Autodesk Inventor part; units mm, degrees
(part 2 of 2)
  line L687 (11.384, -26.5017) -> (12.8968, -23.7765)
  line L688 (8.2674, -26.5542) -> (11.384, -26.5017)
  line L689 (24.5423, -12.481) -> (26.7401, -16.1439)
  line L690 (24.5423, -12.481) -> (20.2713, -12.5528)
  line L691 (24.6668, -19.8787) -> (26.7401, -16.1439)
  line L692 (24.6668, -19.8787) -> (20.3957, -19.9505)
  line L693 (25.5855, -16.1633) -> (24.0727, -18.8885)
  line L694 (24.0727, -18.8885) -> (20.9562, -18.9409)
  line L695 (23.9819, -13.4905) -> (25.5855, -16.1633)
  line L696 (19.3525, -16.2682) -> (20.8654, -13.543)
  line L697 (20.8654, -13.543) -> (23.9819, -13.4905)
  line L698 (20.9562, -18.9409) -> (19.3525, -16.2682)
  line L699 (18.198, -16.2876) -> (20.3957, -19.9505)
  line L700 (20.5202, -27.3482) -> (24.7912, -27.2763)
  line L701 (20.5202, -27.3482) -> (18.3224, -23.6853)
  line L702 (19.4769, -23.6659) -> (21.0806, -26.3386)
  line L703 (20.9898, -20.9407) -> (19.4769, -23.6659)
  line L704 (18.3224, -23.6853) -> (20.3957, -19.9505)
  line L705 (24.1063, -20.8882) -> (20.9898, -20.9407)
  line L706 (25.71, -23.561) -> (24.1063, -20.8882)
  line L707 (24.6668, -19.8787) -> (26.8645, -23.5416)
  line L708 (24.7912, -27.2763) -> (26.8645, -23.5416)
  line L709 (24.1971, -26.2862) -> (25.71, -23.561)
  line L710 (21.0806, -26.3386) -> (24.1971, -26.2862)
  line L711 (30.8867, -8.6744) -> (33.0844, -12.3373)
  line L712 (30.8867, -8.6744) -> (26.6156, -8.7462)
  line L713 (31.0111, -16.072) -> (33.0844, -12.3373)
  line L714 (30.3262, -9.6839) -> (27.2097, -9.7364)
  line L715 (30.3262, -9.6839) -> (31.9299, -12.3567)
  line L716 (30.417, -15.0819) -> (31.9299, -12.3567)
  line L717 (31.0111, -16.072) -> (26.7401, -16.1439)
  line L718 (27.3005, -15.1343) -> (30.417, -15.0819)
  line L719 (26.7401, -16.1439) -> (24.5423, -12.481)
  line L720 (25.6969, -12.4616) -> (27.3005, -15.1343)
  line L721 (25.6969, -12.4616) -> (27.2097, -9.7364)
  line L722 (24.6668, -19.8787) -> (26.8645, -23.5416)
  line L723 (24.6668, -19.8787) -> (26.7401, -16.1439)
  line L724 (25.8213, -19.8592) -> (27.425, -22.532)
  line L725 (25.8213, -19.8592) -> (27.3342, -17.134)
  line L726 (27.3342, -17.134) -> (30.4507, -17.0816)
  line L727 (30.4507, -17.0816) -> (32.0543, -19.7544)
  line L728 (31.0111, -16.072) -> (33.2089, -19.735)
  line L729 (31.1356, -23.4697) -> (33.2089, -19.735)
  line L730 (30.5415, -22.4796) -> (32.0543, -19.7544)
  line L731 (30.5415, -22.4796) -> (27.425, -22.532)
  line L732 (31.1356, -23.4697) -> (26.8645, -23.5416)
  line L733 (37.231, -4.8677) -> (32.96, -4.9396)
  line L734 (37.231, -4.8677) -> (39.4288, -8.5307)
  line L735 (36.6706, -5.8773) -> (38.2742, -8.5501)
  line L736 (36.7614, -11.2753) -> (38.2742, -8.5501)
  line L737 (39.4288, -8.5307) -> (37.3555, -12.2654)
  line L738 (32.0412, -8.6549) -> (33.6449, -11.3277)
  line L739 (33.5541, -5.9297) -> (36.6706, -5.8773)
  line L740 (32.0412, -8.6549) -> (33.5541, -5.9297)
  line L741 (36.7614, -11.2753) -> (33.6449, -11.3277)
  line L742 (37.3555, -12.2654) -> (33.0844, -12.3373)
  line L743 (30.8867, -8.6744) -> (33.0844, -12.3373)
  line L744 (37.4799, -19.6631) -> (39.5532, -15.9283)
  line L745 (37.4799, -19.6631) -> (33.2089, -19.735)
  line L746 (36.8858, -18.673) -> (38.3987, -15.9478)
  line L747 (36.8858, -18.673) -> (33.7693, -18.7254)
  line L748 (33.7693, -18.7254) -> (32.1657, -16.0526)
  line L749 (31.0111, -16.072) -> (33.2089, -19.735)
  line L750 (32.1657, -16.0526) -> (33.6785, -13.3274)
  line L751 (37.3555, -12.2654) -> (33.0844, -12.3373)
  line L752 (36.795, -13.275) -> (33.6785, -13.3274)
  line L753 (36.795, -13.275) -> (38.3987, -15.9478)
  line L754 (37.3555, -12.2654) -> (39.5532, -15.9283)
  line L755 (31.1356, -23.4697) -> (33.3333, -27.1326)
  line L756 (37.6044, -27.0608) -> (33.3333, -27.1326)
  line L757 (32.2901, -23.4503) -> (33.8938, -26.1231)
  line L758 (33.803, -20.7251) -> (32.2901, -23.4503)
  line L759 (31.1356, -23.4697) -> (33.2089, -19.735)
  line L760 (36.9195, -20.6727) -> (33.803, -20.7251)
  line L761 (36.9195, -20.6727) -> (38.5231, -23.3455)
  line L762 (37.4799, -19.6631) -> (39.6777, -23.326)
  line L763 (37.6044, -27.0608) -> (39.6777, -23.326)
  line L764 (37.0103, -26.0706) -> (38.5231, -23.3455)
  line L765 (37.0103, -26.0706) -> (33.8938, -26.1231)
  line L766 (45.8976, -12.1217) -> (43.6998, -8.4588)
  line L767 (45.8976, -12.1217) -> (43.8243, -15.8565)
  line L768 (43.8243, -15.8565) -> (39.5532, -15.9283)
  line L769 (43.2302, -14.8663) -> (44.743, -12.1412)
  line L770 (43.2302, -14.8663) -> (40.1137, -14.9188)
  line L771 (38.51, -12.246) -> (40.1137, -14.9188)
  line L772 (37.3555, -12.2654) -> (39.5532, -15.9283)
  line L773 (38.51, -12.246) -> (40.0229, -9.5208)
  line L774 (43.6998, -8.4588) -> (39.4288, -8.5307)
  line L775 (43.1394, -9.4684) -> (40.0229, -9.5208)
  line L776 (44.743, -12.1412) -> (43.1394, -9.4684)
  line L777 (43.6998, -8.4588) -> (45.8976, -12.1217)
  line L778 (43.9487, -23.2542) -> (39.6777, -23.326)
  line L779 (39.6777, -23.326) -> (37.4799, -19.6631)
  line L780 (37.4799, -19.6631) -> (39.5532, -15.9283)
  line L781 (38.6345, -19.6437) -> (40.2381, -22.3165)
  line L782 (38.6345, -19.6437) -> (40.1473, -16.9185)
  line L783 (43.2638, -16.8661) -> (40.1473, -16.9185)
  line L784 (43.2638, -16.8661) -> (44.8675, -19.5388)
  line L785 (46.022, -19.5194) -> (43.8243, -15.8565)
  line L786 (43.9487, -23.2542) -> (46.022, -19.5194)
  line L787 (44.8675, -19.5388) -> (43.3546, -22.264)
  line L788 (43.3546, -22.264) -> (40.2381, -22.3165)
  line L789 (50.1686, -12.0499) -> (52.2419, -8.3151)
  line L790 (52.2419, -8.3151) -> (50.0442, -4.6522)
  line L791 (49.5745, -11.0597) -> (51.0874, -8.3345)
  line L792 (49.4837, -5.6618) -> (51.0874, -8.3345)
  line L793 (45.7731, -4.724) -> (50.0442, -4.6522)
  line L794 (49.4837, -5.6618) -> (46.3672, -5.7142)
  line L795 (44.8544, -8.4394) -> (46.3672, -5.7142)
  line L796 (46.458, -11.1122) -> (44.8544, -8.4394)
  line L797 (43.6998, -8.4588) -> (45.8976, -12.1217)
  line L798 (49.5745, -11.0597) -> (46.458, -11.1122)
  line L799 (45.8976, -12.1217) -> (50.1686, -12.0499)
  line L800 (46.022, -19.5194) -> (50.2931, -19.4476)
  line L801 (46.022, -19.5194) -> (43.8243, -15.8565)
  line L802 (43.8243, -15.8565) -> (45.8976, -12.1217)
  line L803 (44.9788, -15.8371) -> (46.5825, -18.5098)
  line L804 (46.4917, -13.1119) -> (44.9788, -15.8371)
  line L805 (49.6082, -13.0595) -> (46.4917, -13.1119)
  line L806 (49.6082, -13.0595) -> (51.2119, -15.7322)
  line L807 (50.1686, -12.0499) -> (52.3664, -15.7128)
  line L808 (52.3664, -15.7128) -> (50.2931, -19.4476)
  line L809 (49.699, -18.4574) -> (51.2119, -15.7322)
  line L810 (49.699, -18.4574) -> (46.5825, -18.5098)
  line L811 (46.1465, -26.9171) -> (43.9487, -23.2542)
  line L812 (46.022, -19.5194) -> (43.9487, -23.2542)
  line L813 (46.1465, -26.9171) -> (50.4175, -26.8452)
  line L814 (49.7326, -20.4571) -> (46.6161, -20.5096)
  line L815 (45.1033, -23.2348) -> (46.6161, -20.5096)
  line L816 (46.7069, -25.9075) -> (45.1033, -23.2348)
  line L817 (49.8234, -25.8551) -> (46.7069, -25.9075)
  line L818 (49.8234, -25.8551) -> (51.3363, -23.1299)
  line L819 (50.4175, -26.8452) -> (52.4908, -23.1105)
  line L820 (49.7326, -20.4571) -> (51.3363, -23.1299)
  line L821 (52.4908, -23.1105) -> (50.2931, -19.4476)
  line L822 (50.2931, -19.4476) -> (52.4908, -23.1105)
  line L823 (50.1686, -12.0499) -> (52.2419, -8.3151)
  line L824 (52.2419, -8.3151) -> (50.0442, -4.6522)
  line L825 (52.8024, -7.3055) -> (55.9189, -7.2531)
  line L826 (56.513, -8.2433) -> (52.2419, -8.3151)
  line L827 (52.8024, -7.3055) -> (51.1987, -4.6328)
  line L828 (52.836, -9.3053) -> (51.3232, -12.0305)
  line L829 (55.9525, -9.2528) -> (52.836, -9.3053)
  line L830 (57.5562, -11.9256) -> (55.9525, -9.2528)
  line L831 (56.513, -8.2433) -> (58.7107, -11.9062)
  line L832 (51.3232, -12.0305) -> (52.9268, -14.7032)
  line L833 (50.1686, -12.0499) -> (52.3664, -15.7128)
  line L834 (56.0434, -14.6508) -> (57.5562, -11.9256)
  line L835 (56.6374, -15.6409) -> (58.7107, -11.9062)
  line L836 (56.6374, -15.6409) -> (58.7107, -11.9062)
  line L837 (52.9605, -16.7029) -> (51.4476, -19.4281)
  line L838 (52.3664, -15.7128) -> (50.2931, -19.4476)
  line L839 (56.077, -16.6505) -> (52.9605, -16.7029)
  line L840 (52.9268, -14.7032) -> (56.0434, -14.6508)
  line L841 (56.6374, -15.6409) -> (52.3664, -15.7128)
  line L842 (51.4476, -19.4281) -> (53.0513, -22.1009)
  line L843 (57.6807, -19.3233) -> (56.077, -16.6505)
  line L844 (58.8352, -19.3039) -> (56.6374, -15.6409)
  line L845 (56.1678, -22.0485) -> (57.6807, -19.3233)
  line L846 (56.7619, -23.0386) -> (58.8352, -19.3039)
  line L847 (53.0513, -22.1009) -> (56.1678, -22.0485)
  line L848 (56.513, -8.2433) -> (58.5863, -4.5085)
  line L849 (55.9189, -7.2531) -> (57.4318, -4.5279)
  line L850 (58.5863, -4.5085) -> (56.3885, -0.8456)
  line L851 (57.4318, -4.5279) -> (55.8281, -1.8552)
  line L852 (52.7116, -1.9076) -> (55.8281, -1.8552)
  line L853 (51.1987, -4.6328) -> (52.7116, -1.9076)
  line L854 (50.0442, -4.6522) -> (52.1175, -0.9174)
  line L855 (56.7619, -23.0386) -> (52.4908, -23.1105)
  line L856 (59.2712, -10.8966) -> (57.6675, -8.2238)
  line L857 (56.513, -8.2433) -> (58.7107, -11.9062)
  line L858 (62.4214, -12.8439) -> (59.3048, -12.8963)
  line L859 (58.7107, -11.9062) -> (62.9205, -11.8718)
  line L860 (62.3877, -10.8442) -> (59.2712, -10.8966)
  line L861 (64.1363, -11.8149) -> (65.74, -14.4877)
  line L862 (64.025, -15.5167) -> (62.4214, -12.8439)
  line L863 (62.9205, -11.8718) -> (65.1795, -15.4973)
  line L864 (56.6374, -15.6409) -> (58.7107, -11.9062)
  line L865 (59.3048, -12.8963) -> (57.792, -15.6215)
  line L866 (62.5122, -18.2419) -> (64.025, -15.5167)
  line L867 (59.3956, -18.2943) -> (62.5122, -18.2419)
  line L868 (63.1062, -19.232) -> (58.8352, -19.3039)
  line L869 (57.792, -15.6215) -> (59.3956, -18.2943)
  line L870 (65.1795, -15.4973) -> (63.1062, -19.232)
  line L871 (58.8352, -19.3039) -> (56.6374, -15.6409)
  line L872 (56.7619, -23.0386) -> (58.8352, -19.3039)
  line L873 (69.4506, -15.4254) -> (65.1795, -15.4973)
  line L874 (68.8565, -14.4353) -> (65.74, -14.4877)
  line L875 (64.1363, -11.8149) -> (65.6492, -9.0897)
  line L876 (65.6492, -9.0897) -> (68.7657, -9.0373)
  line L877 (70.3694, -11.7101) -> (68.7657, -9.0373)
  line L878 (68.8565, -14.4353) -> (70.3694, -11.7101)
  line L879 (71.5239, -11.6906) -> (69.4506, -15.4254)
  line L880 (69.3262, -8.0277) -> (71.5239, -11.6906)
  line L881 (69.3262, -8.0277) -> (65.0551, -8.0996)
  line L882 (63.9006, -8.119) -> (62.3877, -10.8442)
  line L883 (65.0551, -8.0996) -> (62.8574, -4.4367)
  line L884 (62.2969, -5.4462) -> (63.9006, -8.119)
  line L885 (62.8574, -4.4367) -> (58.5863, -4.5085)
  line L886 (59.1804, -5.4986) -> (62.2969, -5.4462)
  line L887 (57.6675, -8.2238) -> (59.1804, -5.4986)
  line L888 (56.513, -8.2433) -> (58.5863, -4.5085)
  line L889 (58.9596, -26.7015) -> (56.7619, -23.0386)
  line L890 (58.9596, -26.7015) -> (63.2307, -26.6297)
  line L891 (59.4293, -20.294) -> (62.5458, -20.2416)
  line L892 (57.9164, -23.0192) -> (59.4293, -20.294)
  line L893 (59.5201, -25.692) -> (57.9164, -23.0192)
  line L894 (64.1495, -22.9144) -> (62.6366, -25.6396)
  line L895 (62.6366, -25.6396) -> (59.5201, -25.692)
  line L896 (62.5458, -20.2416) -> (64.1495, -22.9144)
  line L897 (63.1062, -19.232) -> (65.304, -22.8949)
  line L898 (68.6413, -1.6396) -> (70.2449, -4.3124)
  line L899 (70.2449, -4.3124) -> (68.7321, -7.0376)
  line L900 (69.3262, -8.0277) -> (71.3995, -4.293)
  line L901 (65.6156, -7.09) -> (68.7321, -7.0376)
  line L902 (64.0119, -4.4172) -> (65.6156, -7.09)
  line L903 (65.0551, -8.0996) -> (62.8574, -4.4367)
  line L904 (64.0119, -4.4172) -> (65.5247, -1.692)
  line L905 (62.8574, -4.4367) -> (64.9307, -0.7019)
  line L906 (68.6413, -1.6396) -> (65.5247, -1.692)
  line L907 (71.3995, -4.293) -> (69.2017, -0.63)
  line L908 (65.8644, -21.8854) -> (68.981, -21.8329)
  line L909 (69.575, -22.8231) -> (65.304, -22.8949)
  line L910 (64.2608, -19.2126) -> (65.8644, -21.8854)
  line L911 (65.304, -22.8949) -> (63.1062, -19.232)
  line L912 (63.1062, -19.232) -> (65.1795, -15.4973)
  line L913 (64.2608, -19.2126) -> (65.7736, -16.4874)
  line L914 (68.8902, -16.435) -> (65.7736, -16.4874)
  line L915 (71.6484, -19.0883) -> (69.4506, -15.4254)
  line L916 (68.8902, -16.435) -> (70.4938, -19.1077)
  line L917 (70.4938, -19.1077) -> (68.981, -21.8329)
  line L918 (69.575, -22.8231) -> (71.6484, -19.0883)
  line L919 (65.8981, -23.8851) -> (69.0146, -23.8327)
  line L920 (63.2307, -26.6297) -> (65.304, -22.8949)
  line L921 (62.9205, -11.8718) -> (65.0551, -8.0996)
  line L922 (59.1467, -3.4989) -> (57.5431, -0.8262)
  line L923 (56.3885, -0.8456) -> (58.5863, -4.5085)
  line L924 (58.5863, -4.5085) -> (62.8574, -4.4367)
  line L925 (62.2633, -3.4465) -> (59.1467, -3.4989)
  line L926 (64.9307, -0.7019) -> (62.8574, -4.4367)
  line L927 (63.7761, -0.7213) -> (62.2633, -3.4465)
  line L928 (64.9307, -0.7019) -> (62.7329, 2.961)
  line L929 (62.1725, 1.9515) -> (63.7761, -0.7213)
  line L930 (59.0559, 1.899) -> (62.1725, 1.9515)
  line L931 (57.5431, -0.8262) -> (59.0559, 1.899)
  line L932 (56.3885, -0.8456) -> (58.4619, 2.8892)
  line L933 (64.9307, -0.7019) -> (62.7329, 2.961)
  arc A0 (0.2763, 33.2091) -> (0.8367, 34.2186) centre (-0.3178, 34.1992) ccw
  line L934 (4.5137, 35.2806) -> (6.7114, 31.6177)
  line L935 (4.5137, 35.2806) -> (0.2426, 35.2088)
  line L936 (-1.8307, 31.474) -> (0.2426, 35.2088)
  line L937 (5.5569, 31.5983) -> (3.9532, 34.2711)
  line L938 (4.044, 28.8731) -> (5.5569, 31.5983)
  line L939 (6.7114, 31.6177) -> (4.6381, 27.883)
  line L940 (0.9275, 28.8207) -> (4.044, 28.8731)
  line L941 (0.3671, 27.8111) -> (-1.8307, 31.474)
  line L942 (-0.6761, 31.4934) -> (0.9275, 28.8207)
  line L943 (0.8367, 34.2186) -> (-0.6761, 31.4934)
  line L944 (3.9532, 34.2711) -> (0.8367, 34.2186)
  line L945 (13.4291, 13.2313) -> (17.7008, 13.2313)
  line L946 (69.575, -22.8231) -> (71.7728, -26.486)
  line L947 (75.4498, -25.424) -> (72.3332, -25.4764)
  line L948 (76.0439, -26.4142) -> (71.7728, -26.486)
  line L949 (72.3332, -25.4764) -> (70.7296, -22.8037)
  line L950 (72.2424, -20.0785) -> (70.7296, -22.8037)
  line L951 (75.359, -20.026) -> (72.2424, -20.0785)
  line L952 (71.6484, -19.0883) -> (75.9194, -19.0165)
  line L953 (75.359, -20.026) -> (76.9626, -22.6988)
  line L954 (75.9194, -19.0165) -> (78.1172, -22.6794)
  line L955 (75.4498, -25.424) -> (76.9626, -22.6988)
  line L956 (78.1172, -22.6794) -> (76.0439, -26.4142)
  line L957 (75.9194, -19.0165) -> (77.9927, -15.2817)
  line L958 (75.2345, -12.6284) -> (76.8382, -15.3011)
  line L959 (75.795, -11.6188) -> (77.9927, -15.2817)
  line L960 (76.8382, -15.3011) -> (75.3253, -18.0263)
  line L961 (72.2088, -18.0787) -> (75.3253, -18.0263)
  line L962 (75.9194, -19.0165) -> (71.6484, -19.0883)
  line L963 (70.6051, -15.406) -> (72.2088, -18.0787)
  line L964 (70.6051, -15.406) -> (72.118, -12.6808)
  line L965 (69.4506, -15.4254) -> (71.5239, -11.6906)
  line L966 (75.2345, -12.6284) -> (72.118, -12.6808)
  line L967 (71.5239, -11.6906) -> (75.795, -11.6188)
  line L968 (69.2017, -0.63) -> (71.3995, -4.293)
  line L969 (71.3995, -4.293) -> (69.3262, -8.0277)
  line L970 (71.5239, -11.6906) -> (69.3262, -8.0277)
  line L971 (71.9599, -3.2834) -> (70.3562, -0.6106)
  line L972 (71.8691, 2.1146) -> (70.3562, -0.6106)
  line L973 (69.2017, -0.63) -> (71.275, 3.1047)
  line L974 (74.9856, 2.167) -> (71.8691, 2.1146)
  line L975 (75.5461, 3.1766) -> (71.275, 3.1047)
  line L976 (77.7438, -0.4863) -> (75.5461, 3.1766)
  line L977 (74.9856, 2.167) -> (76.5893, -0.5058)
  line L978 (75.0764, -3.231) -> (76.5893, -0.5058)
  line L979 (75.6705, -4.2211) -> (77.7438, -0.4863)
  line L980 (75.0764, -3.231) -> (71.9599, -3.2834)
  line L981 (70.4807, -8.0083) -> (71.9935, -5.2831)
  line L982 (70.4807, -8.0083) -> (72.0844, -10.6811)
  line L983 (75.2009, -10.6286) -> (72.0844, -10.6811)
  line L984 (75.2009, -10.6286) -> (76.7137, -7.9034)
  line L985 (75.795, -11.6188) -> (77.8683, -7.884)
  line L986 (75.6705, -4.2211) -> (77.8683, -7.884)
  line L987 (76.7137, -7.9034) -> (75.1101, -5.2307)
  line L988 (71.9935, -5.2831) -> (75.1101, -5.2307)
  line L989 (75.6705, -4.2211) -> (71.3995, -4.293)
  line L990 (68.7039, 28.9607) -> (70.9017, 25.2978)
  line L991 (70.9017, 25.2978) -> (68.8284, 21.563)
  line L992 (68.9528, 14.1653) -> (71.0261, 17.9001)
  line L993 (68.9528, 14.1653) -> (71.1506, 10.5024)
  line L994 (71.1506, 10.5024) -> (69.0773, 6.7676)
  line L995 (71.4621, 26.3073) -> (69.8585, 28.9801)
  line L996 (71.3713, 31.7053) -> (69.8585, 28.9801)
  line L997 (68.7039, 28.9607) -> (70.7772, 32.6955)
  line L998 (74.4878, 31.7577) -> (71.3713, 31.7053)
  line L999 (75.0483, 32.7673) -> (70.7772, 32.6955)
  line L1000 (77.246, 29.1044) -> (75.0483, 32.7673)
  line L1001 (74.4878, 31.7577) -> (76.0915, 29.085)
  line L1002 (74.5786, 26.3598) -> (76.0915, 29.085)
  line L1003 (75.1727, 25.3696) -> (77.246, 29.1044)
  line L1004 (70.9017, 25.2978) -> (75.1727, 25.3696)
  line L1005 (74.5786, 26.3598) -> (71.4621, 26.3073)
  line L1006 (69.9829, 21.5824) -> (71.4958, 24.3076)
  line L1007 (69.9829, 21.5824) -> (71.5866, 18.9097)
  line L1008 (68.8284, 21.563) -> (71.0261, 17.9001)
  line L1009 (71.0261, 17.9001) -> (75.2972, 17.9719)
  line L1010 (74.7031, 18.9621) -> (71.5866, 18.9097)
  line L1011 (74.7031, 18.9621) -> (76.2159, 21.6873)
  line L1012 (75.2972, 17.9719) -> (77.3705, 21.7067)
  line L1013 (75.1727, 25.3696) -> (77.3705, 21.7067)
  line L1014 (76.2159, 21.6873) -> (74.6123, 24.3601)
  line L1015 (71.4958, 24.3076) -> (74.6123, 24.3601)
  line L1016 (74.7367, 16.9624) -> (71.6202, 16.9099)
  line L1017 (70.1074, 14.1847) -> (71.6202, 16.9099)
  line L1018 (70.1074, 14.1847) -> (71.711, 11.512)
  line L1019 (75.4216, 10.5743) -> (71.1506, 10.5024)
  line L1020 (71.711, 11.512) -> (74.8275, 11.5644)
  line L1021 (71.7447, 9.5123) -> (70.2318, 6.7871)
  line L1022 (74.8612, 9.5647) -> (71.7447, 9.5123)
  line L1023 (69.0773, 6.7676) -> (71.275, 3.1047)
  line L1024 (71.8355, 4.1143) -> (70.2318, 6.7871)
  line L1025 (74.952, 4.1667) -> (71.8355, 4.1143)
  line L1026 (77.6194, 6.9113) -> (75.5461, 3.1766)
  line L1027 (74.952, 4.1667) -> (76.4648, 6.8919)
  line L1028 (74.8612, 9.5647) -> (76.4648, 6.8919)
  line L1029 (75.4216, 10.5743) -> (77.6194, 6.9113)
  line L1030 (75.4216, 10.5743) -> (77.4949, 14.309)
  line L1031 (76.3404, 14.2896) -> (74.8275, 11.5644)
  line L1032 (74.7367, 16.9624) -> (76.3404, 14.2896)
  line L1033 (75.2972, 17.9719) -> (77.4949, 14.309)
  arc A1 (76.7361, 15.7112) -> (76.7361, -6.1888) centre (85.0764, 4.7612) ccw projected
  line L1034 (75.2361, -4.8633) -> (75.2361, -20.6888) projected
  line L1035 (75.2361, 30.2112) -> (75.2361, 14.3857) projected
  arc A2 (76.7361, 15.7112) -> (75.2361, 14.3857) centre (85.0764, 4.7612) ccw projected
  arc A3 (75.2361, 14.3857) -> (75.2361, -4.8633) centre (85.0764, 4.7612) ccw projected
  arc A4 (75.2361, 14.3857) -> (75.2361, -4.8633) centre (85.0764, 4.7612) ccw
  arc A5 (75.2361, 16.8857) -> (75.2361, -7.3633) centre (83.3272, 4.7612) ccw
  line L1036 (75.2361, 16.8857) -> (75.2361, 14.3857)
  line L1037 (75.2361, -4.8633) -> (75.2361, -7.3633)
  line L1038 (75.2361, -4.8633) -> (75.2361, -20.6888) projected
  arc A6 (73.2361, -22.6888) -> (75.2361, -20.6888) centre (73.2361, -20.6888) ccw projected
  line L1039 (73.2361, -22.6888) -> (-9.1639, -22.6888) projected
  line L1040 (73.2361, -22.6888) -> (-9.1639, -22.6888)
  arc A7 (-9.1639, 32.2112) -> (-11.1639, 30.2112) centre (-9.1639, 30.2112) ccw projected
  line L1041 (-9.1639, 32.2112) -> (73.2361, 32.2112)
  line L1042 (61.1217, 15.0112) -> (61.1217, -5.4888) projected
  line L1043 (61.1217, 15.0112) -> (61.1217, -5.4888)
  arc A8 (-9.1639, 32.2112) -> (-11.1639, 30.2112) centre (-9.1639, 30.2112) ccw
  line L1044 (-11.1639, 28.2928) -> (-11.1639, 30.2112)
  arc A9 (-11.1639, -20.6888) -> (-9.1639, -22.6888) centre (-9.1639, -20.6888) ccw projected
  line L1045 (-11.1639, -20.6888) -> (-11.1639, 30.2112)
  arc A10 (-11.1639, -20.6888) -> (-9.1639, -22.6888) centre (-9.1639, -20.6888) ccw
  line L1046 (-6.3851, -20.401) -> (-7.6552, -22.6888)
  line L1047 (4.7626, 20.4853) -> (6.9603, 16.8224)
  line L1048 (-1.5818, 16.6787) -> (0.4915, 20.4134)
  line L1049 (4.887, 13.0876) -> (6.9603, 16.8224)
  line L1050 (5.8058, 16.8029) -> (4.2021, 19.4757)
  line L1051 (4.2929, 14.0777) -> (5.8058, 16.8029)
  line L1052 (4.887, 13.0876) -> (0.616, 13.0157)
  line L1053 (1.1764, 14.0253) -> (4.2929, 14.0777)
  line L1054 (0.616, 13.0157) -> (-1.5818, 16.6787)
  line L1055 (-0.4273, 16.6981) -> (1.1764, 14.0253)
  line L1056 (1.0856, 19.4233) -> (-0.4273, 16.6981)
  line L1057 (4.2021, 19.4757) -> (1.0856, 19.4233)
  line L1058 (-8.175, 27.6674) -> (-6.1017, 31.4022)
  line L1059 (-8.175, 27.6674) -> (-5.9773, 24.0045)
  line L1060 (-1.7062, 24.0763) -> (-5.9773, 24.0045)
  line L1061 (-5.5076, 30.412) -> (-7.0205, 27.6868)
  line L1062 (-2.3911, 30.4644) -> (-5.5076, 30.412)
  line L1063 (-6.1017, 31.4022) -> (-1.8307, 31.474)
  line L1064 (-1.8307, 31.474) -> (0.3671, 27.8111)
  line L1065 (-0.7875, 27.7917) -> (-2.3911, 30.4644)
  line L1066 (-2.3003, 25.0665) -> (-0.7875, 27.7917)
  line L1067 (-5.4168, 25.0141) -> (-2.3003, 25.0665)
  line L1068 (-7.0205, 27.6868) -> (-5.4168, 25.0141)
  line L1069 (-12.5705, 34.9932) -> (-14.6438, 31.2585)
  line L1070 (-12.5705, 34.9932) -> (-8.2995, 35.0651)
  line L1071 (-13.4893, 31.2779) -> (-11.9765, 34.0031)
  line L1072 (-11.9765, 34.0031) -> (-8.8599, 34.0555)
  line L1073 (-6.1017, 31.4022) -> (-8.2995, 35.0651)
  line L1074 (-8.8599, 34.0555) -> (-7.2563, 31.3827)
  line L1075 (-7.2563, 31.3827) -> (-8.7691, 28.6576)
  line L1076 (-8.7691, 28.6576) -> (-11.8856, 28.6051)
  line L1077 (-8.175, 27.6674) -> (-12.4461, 27.5956)
  line L1078 (-11.8856, 28.6051) -> (-13.4893, 31.2779)
  line L1079 (-14.6438, 31.2585) -> (-12.4461, 27.5956)
  line L1080 (0.4915, 20.4134) -> (-1.7062, 24.0763)
  line L1081 (0.4915, 20.4134) -> (-1.5818, 16.6787)
  line L1082 (-2.2667, 23.0668) -> (-0.663, 20.394)
  line L1083 (-0.663, 20.394) -> (-2.1759, 17.6688)
  line L1084 (-5.8528, 16.6068) -> (-1.5818, 16.6787)
  line L1085 (-2.1759, 17.6688) -> (-5.2924, 17.6164)
  line L1086 (-8.0506, 20.2697) -> (-5.8528, 16.6068)
  line L1087 (-5.2924, 17.6164) -> (-6.8961, 20.2891)
  line L1088 (-6.8961, 20.2891) -> (-5.3832, 23.0143)
  line L1089 (-8.0506, 20.2697) -> (-5.9773, 24.0045)
  line L1090 (-5.3832, 23.0143) -> (-2.2667, 23.0668)
  line L1091 (-12.3216, 20.1979) -> (-8.0506, 20.2697)
  line L1092 (-12.3216, 20.1979) -> (-14.5194, 23.8608)
  line L1093 (-8.6447, 21.2599) -> (-11.7612, 21.2074)
  line L1094 (-11.7612, 21.2074) -> (-13.3649, 23.8802)
  line L1095 (-12.4461, 27.5956) -> (-14.5194, 23.8608)
  line L1096 (-13.3649, 23.8802) -> (-11.852, 26.6054)
  line L1097 (-8.175, 27.6674) -> (-12.4461, 27.5956)
  line L1098 (-11.852, 26.6054) -> (-8.7355, 26.6578)
  line L1099 (-8.7355, 26.6578) -> (-7.1318, 23.9851)
  line L1100 (-7.1318, 23.9851) -> (-8.6447, 21.2599)
  line L1101 (-8.0506, 20.2697) -> (-5.9773, 24.0045)
  line L1102 (-14.395, 16.4631) -> (-12.1972, 12.8002)
  line L1103 (-7.9261, 12.872) -> (-12.1972, 12.8002)
  line L1104 (-14.395, 16.4631) -> (-12.3216, 20.1979)
  line L1105 (-8.0506, 20.2697) -> (-12.3216, 20.1979)
  line L1106 (-8.611, 19.2602) -> (-11.7276, 19.2077)
  line L1107 (-7.0074, 16.5874) -> (-8.611, 19.2602)
  line L1108 (-8.5202, 13.8622) -> (-7.0074, 16.5874)
  line L1109 (-5.8528, 16.6068) -> (-7.9261, 12.872)
  line L1110 (-11.6368, 13.8098) -> (-8.5202, 13.8622)
  line L1111 (-13.2404, 16.4825) -> (-11.6368, 13.8098)
  line L1112 (-11.7276, 19.2077) -> (-13.2404, 16.4825)
  arc A11 (25.4631, 15.0112) -> (25.4631, -5.4888) centre (13.8361, 4.7612) ccw projected
  line L1113 (61.1217, -5.4888) -> (25.4631, -5.4888) projected
  line L1114 (25.4631, -5.4888) -> (61.1217, -5.4888)
  arc A12 (26.1217, 16.5112) -> (26.1217, -6.9888) centre (13.8361, 4.7612) ccw projected
  line L1115 (61.1218, -6.9888) -> (26.1217, -6.9888)
  line L1116 (62.6217, -6.9888) -> (62.6217, 16.5112)
  line L1117 (61.1218, -6.9888) -> (62.6217, -6.9888)
  line L1118 (26.1217, 16.5112) -> (60.6217, 16.5112) projected
  line L1119 (62.6217, 16.5112) -> (26.1217, 16.5112)
  line L1120 (25.4631, 15.0112) -> (61.1217, 15.0112) projected
  line L1121 (-6.6639, -22.6888) -> (-9.1639, -22.6888) projected
  line L1122 (-9.1639, -22.6888) -> (-9.1639, 32.2112)
  arc A13 (-9.1639, 32.2112) -> (-11.1639, 30.2112) centre (-9.1639, 30.2112) ccw projected
  arc A14 (75.2361, 30.2112) -> (73.2361, 32.2112) centre (73.2361, 30.2112) ccw projected
  line L1123 (-11.1639, 30.2112) -> (75.2361, 30.2112)
  line L1124 (-9.1639, 32.2112) -> (73.2361, 32.2112) projected
  line L1125 (73.2361, 32.2112) -> (73.2361, -22.6888)
  line L1126 (75.2361, -20.6888) -> (-11.1639, -20.6888)
  point P0 (0, 0)
  point P1 (-3.2818, -9.2492)
  point P2 (-3.4062, -1.8515)
  point P3 (-3.2818, -9.2492)
  point P4 (-3.4062, -1.8515)
  point P5 (-0.0641, 3.8103)
  point P6 (-3.5306, 5.5462)
  point P7 (-3.6551, 12.9439)
  point P8 (-3.6551, 12.9439)
  point P9 (-0.2984, -0.179)
  point P10 (-13.236, 7.0031)
  point P11 (-9.9995, 9.1373)
  point P12 (-9.9995, 9.1373)
  point P13 (15.5024, 16.9661)
  point P14 (15.5024, 16.9661)
  point P15 (9.0336, 20.5571)
  point P16 (9.0336, 20.5571)
  point P17 (34.7844, 13.5905)
  point P18 (34.7844, 13.5905)
  point P19 (34.6599, 20.9882)
  point P20 (34.6599, 20.9882)
  point P21 (41.0043, 24.7948)
  point P22 (41.0043, 24.7948)
  point P23 (34.5355, 28.3859)
  point P24 (34.5355, 28.3859)
  point P25 (41.1287, 17.3971)
  point P26 (41.1287, 17.3971)
  point P27 (28.6889, -5.0114)
  point P28 (28.6889, -5.0114)
  point P29 (60.4107, 14.0216)
  point P30 (60.4107, 14.0216)
  point P31 (68.3924, 13.1558)
  point P32 (65.2759, 13.1033)
  point P33 (68.4832, 7.7578)
  point P34 (31.419, 28.3335)
  point P35 (37.652, 28.4383)
  point P36 (36.0484, 31.1111)
  point P37 (0.2763, 33.2091)
  point P38 (49.5745, -11.0597)
  point P39 (51.0874, -8.3345)
  point P40 (46.3672, -5.7142)
  point P41 (49.6082, -13.0595)
  point P42 (49.8234, -25.8551)
  point P43 (51.3363, -23.1299)
  point P44 (68.8902, -16.435)
  point P45 (65.7736, -16.4874)
  point P46 (68.981, -21.8329)
  point P47 (68.8565, -14.4353)
  point P48 (68.7657, -9.0373)
  point P49 (65.74, -14.4877)
  point P50 (68.7321, -7.0376)
  point P51 (68.6413, -1.6396)
  point P52 (65.5247, -1.692)
  point P53 (68.5168, 5.7581)
  point P54 (65.4911, 0.3077)
  point P55 (68.6076, 0.3601)
  point P56 (65.2422, 15.103)
  point P57 (68.3587, 15.1555)
  point P58 (68.2679, 20.5534)
  point P59 (64.9933, 29.8984)
  point P60 (68.1098, 29.9508)
  point P61 (68.019, 35.3488)
  point P62 (68.2343, 22.5532)
  point P63 (68.1435, 27.9511)
  point P64 (65.027, 27.8987)
  point P65 (71.6202, 16.9099)
  point P66 (70.1074, 14.1847)
  point P67 (74.8275, 11.5644)
  point P68 (74.5786, 26.3598)
  point P69 (76.0915, 29.085)
  point P70 (69.8585, 28.9801)
  point P71 (69.9829, 21.5824)
  point P72 (71.5866, 18.9097)
  point P73 (74.6123, 24.3601)
  point P74 (76.4648, 6.8919)
  point P75 (74.8612, 9.5647)
  point P76 (70.2318, 6.7871)
  point P77 (70.3562, -0.6106)
  point P78 (76.5893, -0.5058)
  point P79 (75.1101, -5.2307)
  point P80 (70.4807, -8.0083)
  point P81 (72.0844, -10.6811)
  point P82 (72.118, -12.6808)
  point P83 (70.6051, -15.406)
  point P84 (75.3253, -18.0263)
  point P85 (70.7296, -22.8037)
  point P86 (76.9626, -22.6988)
  point P87 (75.359, -20.026)
  point P88 (75.7664, -6.3246)
  point P89 (72.7518, -5.2703)
  point P90 (72.1483, -3.2802)
  point P91 (70.4289, -0.4798)
  point P92 (70.3451, 6.5982)
  point P93 (70.4262, 7.1373)
  point P94 (71.9131, 11.5154)
  point P95 (74.915, 16.6652)
  point P96 (70.9618, -23.1906)
  point P97 (76.0241, -21.1346)
  point P98 (20.0193, -22.6888)
  point P99 (25.1867, -22.6888)
  point P100 (32.7128, -22.6888)
  point P101 (38.1291, -22.6888)
  point P102 (45.4063, -22.6888)
  point P103 (51.3026, -23.1906)
  point P104 (58.0193, -23.1906)
  point P105 (63.9961, -23.1906)
  point P106 (-5.3677, -22.6888)
  point P107 (-0.6983, -22.6888)
  point P108 (7.3258, -22.6888)
  point P109 (12.2442, -22.6888)
  point P110 (31.0741, 32.2112)
  point P111 (25.1093, 32.2112)
  point P112 (43.7777, 32.6094)
  point P113 (37.8028, 32.2112)
  point P114 (56.7202, 32.6094)
  point P115 (50.7173, 32.6094)
  point P116 (69.3647, 32.2112)
  point P117 (63.4109, 32.6094)
  point P118 (5.1891, 32.2112)
  point P119 (-0.2777, 32.2112)
  point P120 (18.1316, 32.2112)
  point P121 (12.4158, 32.2112)
  point P122 (-11.1639, -10.3819)
  point P123 (-11.1005, -15.7803)
  point P124 (-11.1639, -2.9821)
  point P125 (-11.1639, -8.3816)
  point P126 (-11.1639, 4.4177)
  point P127 (-11.1639, -0.9818)
  point P128 (-11.1639, 11.8174)
  point P129 (-11.1639, 6.4179)
  point P130 (-11.1005, -17.7806)
  point P131 (-7.6552, -22.6888)
  point P132 (70.7934, -22.6888)
  point P133 (51.0716, -22.6888)
  point P134 (58.0999, -22.6888)
  point P135 (64.0141, -22.6888)
  point P136 (43.9776, 32.2112)
  point P137 (56.6711, 32.2112)
  point P138 (50.6632, 32.2112)
  point P139 (63.6056, 32.2112)
  point P140 (-11.3324, -10.5679)
  point P141 (-11.1639, -15.7393)
  point P142 (-11.4238, -3.1107)
  point P143 (-11.3324, -8.2683)
  point P144 (-11.4238, -0.9257)
  point P145 (-11.1639, -17.8863)
  point P146 (-7.7534, 32.2112)
  point P147 (-11.1639, 28.6173)
  point P148 (-11.1639, 26.617)
  point P149 (-11.1639, 21.2175)
  point P150 (-11.1639, 19.2172)
  point P151 (-11.1639, 13.8177)
  point P152 (75.2361, 19.9222)
  point P153 (75.2361, 23.3204)
  point P154 (75.5676, -20.3738)
  point P155 (75.2361, -10.5652)
  point P156 (75.2361, -5.4407)
  point P157 (75.5676, -17.5899)
  point P158 (75.2361, -12.6309)
  point P159 (75.2361, 27.544)
  point P160 (75.5676, 29.9581)
  point P161 (75.2361, -20.0281)
  point P162 (75.2361, -18.0278)
  point P163 (71.0484, 12.6163)
  point P164 (75.2361, 16.1301)
  point P165 (-1.4503, 7.3256)
  point P166 (-1.6082, 3.4477)
  point P167 (0.8998, -3.7771)
  point P168 (4.8167, -7.8444)
  point P169 (6.5171, -8.902)
  point P170 (11.7505, -10.5978)
  point P171 (13.96, -10.7383)
  point P172 (17.72, -10.2443)
  point P173 (19.6661, -9.6006)
  point P174 (24.2391, -6.7291)
  point P175 (25.8274, -5.4888)
  point P176 (31.5113, -5.4888)
  point P177 (38.7698, -5.4888)
  point P178 (44.2048, -5.4888)
  point P179 (51.7123, -5.4888)
  point P180 (56.8983, -5.4888)
  point P181 (59.7664, -5.4888)
  point P182 (61.1217, -5.466)
  point P183 (61.1217, -3.4657)
  point P184 (61.1217, 1.9338)
  point P185 (61.1217, 3.9341)
  point P186 (61.1217, 9.3336)
  point P187 (61.1217, 11.3338)
  point P188 (57.8727, 15.0112)
  point P189 (55.5851, 15.0112)
  point P190 (52.3548, 15.0112)
  point P191 (50.0224, 15.0112)
  point P192 (45.1791, 15.0112)
  point P193 (42.8916, 15.0112)
  point P194 (39.4123, 15.0112)
  point P195 (37.08, 15.0112)
  point P196 (32.4856, 15.0112)
  point P197 (21.7783, 18.0718)
  point P198 (19.6959, 19.1109)
  point P199 (11.8886, 20.1384)
  dimension "d253" = 1
  dimension "d257" = 1
  dimension "d261" = 1
  dimension "d264" = 1.5
  dimension "d265" = 1.5
  dimension "d266" = 2.5
  dimension "d267" = 2.5
  constraints: 2232 end point, 925 symmetric about line, 16 coincident, 10 point on circle, 7 horizontal, 5 centre point, 5 point on line, 3 perpendicular, 3 vertical, 2 collinear, 2 concentric, 44 other
  measures "d253" distance between parallel lines of L3 L14
  measures "d257" distance between parallel lines of L43 L44
  measures "d261" distance between parallel lines of L615 L184
  measures "d264" distance between parallel lines of L1116 L1042
  measures "d265" distance between parallel lines of L1120 L1118
  measures "d266" distance of L1035.end L1036.start
  measures "d267" distance of L1037.end L1034.start
extrude "CardBedHex" cut sketch "Sketch21" against normal blind 15.7 contours L184 L185 L182 A12 | L123 L131 L130 L129 L1122 | L1122 L173 L172 L171 L170 | L150 L149 L147 L1126 L1122 | A11 L6 L10 L9 | L9 L48 L45 L180 A11 L183 L186 L181 L182 | L22 L17 L18 L19 L20 A12 | L180 L46 L288 L623 A11 L628 L627 L626 L631 | A12 L629 L630 | L675 L676 L668 L669 L670 L1126 | L10 L27 L26 A11 L1052 L1049 L91 L80 L945 L72 L73 L74 L71 L70 L188 L199 L252 L260 L257 L310 L314 L311 L308 L362 L361 L303 L302 L356 L353 L270 L271 L273 L272 L274 L276 L275 L289 L290 L288 L46 L45 L48 | A11 L32 L33 L26 L27 L6 | L182 L181 L186 L183 A11 | L631 L626 L627 L628 A11 | L1122 L162 L161 L160 L159 | A11 L33 L32 | L623 L290 L291 A11 L649 L647 L655 | A12 L649 L650 L652 L654 L655 | L661 L663 L665 L666 L658 L1126 | L31 L30 L29 L28 A12 | L655 L647 L649 A11 | L1122 L61 L67 L64 L65 | L289 L275 L277 A11 L301 L295 L293 L298 L291 | L35 L36 L43 L40 L41 A12 | A11 L1053 L1051 L1050 L94 L1049 L1052 | A12 L301 L296 L299 L298 | L1122 L1106 L1107 L1108 L1110 | A11 L1050 L1051 L1053 | L276 L274 L272 L284 L1113 L283 L282 L280 L278 L287 A11 L277 | L298 L293 L295 L301 A11 | L724 L725 L726 L727 L730 L1126 | L94 A11 L87 L90 L89 L75 L91 | L1055 L1056 L1057 L1050 A12 | L1122 L1098 L1099 L1100 L1093 | L75 A11 L84 L72 L945 L80 | L1115 L283 L285 L287 | L284 L273 L359 L1113 | L1115 L735 L736 L741 L738 L740 | A11 L89 L90 L87 | L287 L278 L280 L282 L283 L1113 | L359 L271 L270 L353 L355 L1113 L354 L352 L366 L360 L358 | L87 L85 L86 L92 A12 | L1123 L1065 L1066 L1067 L1068 L1061 | A11 L393 L394 L73 L84 | L358 L360 L366 L352 L354 L1113 | L781 L782 L783 L784 L787 L1126 | A11 L394 L393 | L1115 L354 L357 L358 | A12 L421 L422 | L422 L415 L416 L419 L420 L421 A12 | L1123 L453 L452 L450 L449 L451 | L355 L356 L790 L1113 | L1115 L792 L791 L798 L796 L795 | L399 L398 L396 L395 A12 | A11 L1120 L382 L383 L384 L194 L71 L74 | L790 L302 L303 L850 L848 L1113 L849 L851 L852 L853 L827 | L1123 L432 L433 L426 L427 L429 | L827 L853 L852 L851 L849 L1113 | L842 L837 L839 L843 L845 L1126 | L388 L389 L385 L384 L1118 A12 | L194 L1120 L195 L196 L197 L206 L205 L198 L199 L188 L70 | L1120 L384 L383 L382 | L1115 L849 L825 L827 | L361 L317 L1042 L930 L931 L922 L925 L885 L850 | L848 L885 L1042 L886 L1113 | L1115 L1117 L1116 L884 L882 L860 L856 L887 | L1120 L205 L206 L197 L196 L195 | L362 L308 L319 L1042 L320 L307 L328 L316 L317 | L886 L1042 L1113 | L1123 L242 L239 L236 L209 L213 | L198 L1120 L245 L251 L253 L254 L252 | L910 L913 L914 L916 L917 L1126 | L254 L1120 L372 L371 L370 L374 L377 L305 L310 L257 L260 | L245 L255 L248 L250 L253 L1118 | L316 L328 L307 L320 L1042 | L1042 L925 L922 L931 L930 | L311 L332 L1120 L336 L313 L318 L1042 L319 | L1120 L253 L251 L245 | L929 L927 L1116 | L1116 L323 L324 | L314 L305 L1120 L304 L306 L329 L332 | L1120 L377 L374 L370 L371 L372 | L318 L313 L336 L1120 L1042 | L983 L982 L981 L988 A5 L1125 | L1125 L961 L963 L964 L966 | L1123 L514 L513 L517 L518 L519 | L375 L377 L1118 | L329 L306 L304 L1120 | L563 L559 L556 L560 L561 L562 A5 | L347 L326 L321 L343 L344 L346 A5 | L1118 L304 L335 L334 L330 L329 | L336 L338 L339 L1119 L1118 | L1116 L339 L341 | L1123 L537 L544 L543 L541 L540 | L1018 L1017 L1016 L1125 A5 | L1010 L1007 L1006 L1015 L1125 | L1005 L995 L996 L1123 L1125 | L11 L12 L13 L14 L15 L16 | L76 L77 L83 L81 L82 L78 | L120 L119 L118 L117 L116 L115 | L189 L207 L235 L202 L203 L191 | L216 L221 L222 L219 L217 L200 | L227 L230 L232 L231 L229 L226 | L404 L405 L407 L409 L410 L411 | L460 L462 L466 L465 L464 L461 | L523 L532 L531 L528 L527 L525 | L548 L551 L553 L554 L550 L546 | L570 L571 L572 L573 L569 L567 | L581 L583 L584 L586 L587 L580 | L621 L620 L619 L618 L617 L616 | L636 L637 L638 L640 L642 L644 | L693 L694 L698 L696 L697 L695 | L715 L716 L718 L720 L721 L714 | L747 L748 L750 L752 L753 L746 | L770 L771 L773 L775 L776 L769 | L804 L805 L806 L809 L810 L803 | L829 L830 L834 L840 L832 L828 | L862 L866 L867 L869 L865 L858 | L875 L876 L877 L878 L874 L861 | L898 L899 L901 L902 L904 L906 | L1082 L1083 L1085 L1087 L1088 L1090
equation "\"d89\" = d19"
body "Solid3"
